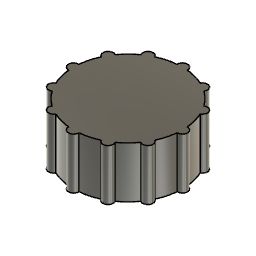
Knob (Autodesk Fusion 360 design; units mm, degrees)
Autodesk Fusion 360 part; units mm, degrees
sketch "Sketch1" plane through (0, 0, 0) normal (0, 0, 1) x (1, 0, 0) in component "Knob"
  circle A0 centre (0, 0) radius 3
  line L0 (-2.5981, 1.5) -> (2.5981, 1.5)
  circle A1 centre (0, 0) radius 16
  circle A2 centre (0, 16) radius 1.5
  circle A3 centre (-8, 13.8564) radius 1.5
  circle A4 centre (-13.8564, 8) radius 1.5
  circle A5 centre (-16, 0) radius 1.5
  circle A6 centre (-13.8564, -8) radius 1.5
  circle A7 centre (-8, -13.8564) radius 1.5
  circle A8 centre (0, -16) radius 1.5
  circle A9 centre (8, -13.8564) radius 1.5
  circle A10 centre (13.8564, -8) radius 1.5
  circle A11 centre (16, 0) radius 1.5
  circle A12 centre (13.8564, 8) radius 1.5
  circle A13 centre (8, 13.8564) radius 1.5
  point P0 (0, -3)
  dimension "d1" = 6
  dimension "d3" = 4.5
  dimension "d4" = 32
  dimension "d5" = 3
  dimension "d7" = 360
  constraint coincident A0.centre A1.centre
  constraint coincident A0 L0.start
  constraint coincident A0 L0.end
  constraint horizontal L0
  constraint coincident A0 P0
  constraint vertical A0.centre P0
  constraint coincident A1 A2.centre
  constraint vertical A0.centre A2.centre
  measures "d1" diameter of A0
  measures "d3" distance of L0 P0
  measures "d4" diameter of A1
  measures "d5" diameter of A2
extrude "Extrude1" add sketch "Sketch1" along normal blind 12 contours A0 L0 | A1 A11 | A1 A11 | A1 A2 A3 A4 A5 A6 A7 A8 A9 A10 A11 A12 A13 | A1 A12 | A1 A12 | A1 A10 | A1 A10 | A1 A13 | A1 A13 | A1 A9 | A1 A9 | A1 A2 | A1 A2 | A1 A8 | A1 A8 | A1 A3 | A1 A3 | A1 A7 | A1 A7 | A1 A4 | A1 A4 | A1 A6 | A1 A6 | A1 A5 | A1 A5 picked at (0.6802, 1.7331) in component "Knob"
extrude "Extrude2" add sketch "Sketch1" along normal blind 3 from surface at 12 contours A0 L0 | A0 L0 | A1 A11 | A1 A11 | A1 A2 A3 A4 A5 A6 A7 A8 A9 A10 A11 A12 A13 | A1 A12 | A1 A12 | A1 A10 | A1 A10 | A1 A13 | A1 A13 | A1 A9 | A1 A9 | A1 A2 | A1 A2 | A1 A8 | A1 A8 | A1 A3 | A1 A3 | A1 A7 | A1 A7 | A1 A4 | A1 A4 | A1 A6 | A1 A6 | A1 A5 | A1 A5 in component "Knob"
sketch "Sketch2" plane through (0, 0, 15) normal (0, 0, 1) x (-1, 0, 0) in component "Knob"
  arc A0 (-9.2625, -13.0463) -> (-6.6672, -14.5447) centre (-8, -13.8564) ccw
  arc A1 (-6.6672, -14.5447) -> (-1.4984, -15.9297) centre (0, 0) ccw
  arc A2 (-1.4984, -15.9297) -> (1.4984, -15.9297) centre (0, -16) ccw
  arc A3 (1.4984, -15.9297) -> (6.6672, -14.5447) centre (0, 0) ccw
  arc A4 (6.6672, -14.5447) -> (9.2625, -13.0463) centre (8, -13.8564) ccw
  arc A5 (9.2625, -13.0463) -> (13.0463, -9.2625) centre (0, 0) ccw
  arc A6 (13.0463, -9.2625) -> (14.5447, -6.6672) centre (13.8564, -8) ccw
  arc A7 (14.5447, -6.6672) -> (15.9297, -1.4984) centre (0, 0) ccw
  arc A8 (15.9297, -1.4984) -> (15.9297, 1.4984) centre (16, 0) ccw
  arc A9 (15.9297, 1.4984) -> (14.5447, 6.6672) centre (0, 0) ccw
  arc A10 (14.5447, 6.6672) -> (13.0463, 9.2625) centre (13.8564, 8) ccw
  arc A11 (13.0463, 9.2625) -> (9.2625, 13.0463) centre (0, 0) ccw
  arc A12 (9.2625, 13.0463) -> (6.6672, 14.5447) centre (8, 13.8564) ccw
  arc A13 (6.6672, 14.5447) -> (1.4984, 15.9297) centre (0, 0) ccw
  arc A14 (1.4984, 15.9297) -> (-1.4984, 15.9297) centre (0, 16) ccw
  arc A15 (-1.4984, 15.9297) -> (-6.6672, 14.5447) centre (0, 0) ccw
  arc A16 (-6.6672, 14.5447) -> (-9.2625, 13.0463) centre (-8, 13.8564) ccw
  arc A17 (-9.2625, 13.0463) -> (-13.0463, 9.2625) centre (0, 0) ccw
  arc A18 (-13.0463, 9.2625) -> (-14.5447, 6.6672) centre (-13.8564, 8) ccw
  arc A19 (-14.5447, 6.6672) -> (-15.9297, 1.4984) centre (0, 0) ccw
  arc A20 (-15.9297, 1.4984) -> (-15.9297, -1.4984) centre (-16, 0) ccw
  arc A21 (-15.9297, -1.4984) -> (-14.5447, -6.6672) centre (0, 0) ccw
  arc A22 (-14.5447, -6.6672) -> (-13.0463, -9.2625) centre (-13.8564, -8) ccw
  arc A23 (-13.0463, -9.2625) -> (-9.2625, -13.0463) centre (0, 0) ccw
  line L0 (0.5, -15) -> (-0.5, -15)
  line L1 (-0.5, -15) -> (-0.5, -4)
  line L2 (-0.5, -4) -> (0.5, -4)
  line L3 (0.5, -4) -> (0.5, -15)
  line L4 (1.567, -3.7141) -> (2.433, -3.2141)
  line L5 (2.433, -3.2141) -> (7.933, -12.7404)
  line L6 (7.067, -13.2404) -> (1.567, -3.7141)
  line L7 (7.933, -12.7404) -> (7.067, -13.2404)
  line L8 (3.2141, -2.433) -> (3.7141, -1.567)
  line L9 (3.7141, -1.567) -> (13.2404, -7.067)
  line L10 (12.7404, -7.933) -> (3.2141, -2.433)
  line L11 (13.2404, -7.067) -> (12.7404, -7.933)
  line L12 (4, -0.5) -> (4, 0.5)
  line L13 (4, 0.5) -> (15, 0.5)
  line L14 (15, -0.5) -> (4, -0.5)
  line L15 (15, 0.5) -> (15, -0.5)
  line L16 (3.7141, 1.567) -> (3.2141, 2.433)
  line L17 (3.2141, 2.433) -> (12.7404, 7.933)
  line L18 (13.2404, 7.067) -> (3.7141, 1.567)
  line L19 (12.7404, 7.933) -> (13.2404, 7.067)
  line L20 (2.433, 3.2141) -> (1.567, 3.7141)
  line L21 (1.567, 3.7141) -> (7.067, 13.2404)
  line L22 (7.933, 12.7404) -> (2.433, 3.2141)
  line L23 (7.067, 13.2404) -> (7.933, 12.7404)
  line L24 (0.5, 4) -> (-0.5, 4)
  line L25 (-0.5, 4) -> (-0.5, 15)
  line L26 (0.5, 15) -> (0.5, 4)
  line L27 (-0.5, 15) -> (0.5, 15)
  line L28 (-1.567, 3.7141) -> (-2.433, 3.2141)
  line L29 (-2.433, 3.2141) -> (-7.933, 12.7404)
  line L30 (-7.067, 13.2404) -> (-1.567, 3.7141)
  line L31 (-7.933, 12.7404) -> (-7.067, 13.2404)
  line L32 (-3.2141, 2.433) -> (-3.7141, 1.567)
  line L33 (-3.7141, 1.567) -> (-13.2404, 7.067)
  line L34 (-12.7404, 7.933) -> (-3.2141, 2.433)
  line L35 (-13.2404, 7.067) -> (-12.7404, 7.933)
  line L36 (-4, 0.5) -> (-4, -0.5)
  line L37 (-4, -0.5) -> (-15, -0.5)
  line L38 (-15, 0.5) -> (-4, 0.5)
  line L39 (-15, -0.5) -> (-15, 0.5)
  line L40 (-3.7141, -1.567) -> (-3.2141, -2.433)
  line L41 (-3.2141, -2.433) -> (-12.7404, -7.933)
  line L42 (-13.2404, -7.067) -> (-3.7141, -1.567)
  line L43 (-12.7404, -7.933) -> (-13.2404, -7.067)
  line L44 (-2.433, -3.2141) -> (-1.567, -3.7141)
  line L45 (-1.567, -3.7141) -> (-7.067, -13.2404)
  line L46 (-7.933, -12.7404) -> (-2.433, -3.2141)
  line L47 (-7.067, -13.2404) -> (-7.933, -12.7404)
  dimension "d18" = 11
  dimension "d19" = 1
  dimension "d20" = 0.5
  dimension "d21" = 4
  dimension "d23" = 360
  constraint horizontal L0
  constraint vertical L1
  constraint horizontal L2
  constraint vertical L3
  measures "d18" distance of L0.end L1.end
  measures "d19" distance of L0.start L0.end
  measures "d20" distance of A1.centre L3
  measures "d21" distance of A1.centre L2
component "Knob" placed x (1, 0, 0) y (0, 1, 0) z (0, 0, 1) at (0, 0, 0)
equation "d20 = d19 / 2"
